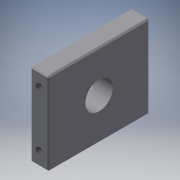
# Autodesk Inventor part: Ramka4
Saved by Autodesk Inventor 2019 (Build 230136000, 136)
## iProperties
Created: 2020-08-21
Part Number: Ramka4
Material: Steel(1)
Document SubType Name: Modeling
Designer: estee
Density: 7.85 g/cm^3
Appearance: Plate(1)
Author: estee
Autodesk Inventor part; units mm, degrees
ref_plane "YZ Plane" through (0, 0, 0) normal (1, 0, 0) x (0, 1, 0)
ref_plane "XZ Plane" through (0, 0, 0) normal (0, 1, 0) x (-1, 0, 0)
ref_plane "XY Plane" through (0, 0, 0) normal (0, 0, 1) x (1, 0, 0)
sketch "Sketch1" plane through (0, 0, 0) normal (1, 0, 0) x (0, 1, 0)
  line L0 (0, 0) -> (-18, 0)
  line L1 (-18, 0) -> (-18, -22)
  line L2 (-18, -22) -> (0, -22)
  line L3 (0, -22) -> (0, 0)
  dimension "d0" = 18
  dimension "d1" = 22
  constraints: 8 end point, 2 parallel, 1 horizontal, 1 perpendicular
  measures "d0" distance of L2.end L1.end
  measures "d1" distance of L2.end L0.start
extrude "Extrusion1" add sketch "Sketch1" along normal blind 4
chamfer "Chamfer1" distance 0.3 angle 45 12 edges at (4, 0, -11) (0, 0, -11) (2, 0, -22) (4, -9, 0) (2, 0, 0) (0, -9, -22) (2, -18, -22) (4, -9, -22) (4, -18, -11) (0, -18, -11) (0, -9, 0) (2, -18, 0)
sketch "Sketch2" plane through (0.3, -17.7, 0) normal (0, 0, 1) x (1, 0, 0)
  line L0 (-0.3, 17.4) -> (-0.3, 0) projected
  line L1 (3.4, 17.7) -> (0, 17.7) projected
  line L2 (0, -0.3) -> (3.4, -0.3) projected
  point P0 (-0.3, 17.7)
  point P1 (1.7, 14.7)
  point P2 (1.7, 2.7)
  dimension "d7" = 2
  dimension "d8" = 2
  dimension "d9" = 3
  dimension "d10" = 3
  measures "d7" distance from line of L0 point (1.7, 14.7)
  measures "d8" distance from line of L0 point (1.7, 2.7)
  measures "d9" distance from line of L1 point (1.7, 14.7)
  measures "d10" distance from line of L2 point (1.7, 2.7)
hole "Hole1" at (2, -3, 0) at (2, -15, 0) direction (0, 0, -1) diameter 1.567 depth 6.3 tip angle 118 thread size "M2x0.4" class "6H" standard "ISO Metric profile"
sketch "Sketch3" plane through (3.7, -17.7, -22) normal (0, 0, -1) x (-1, 0, 0)
  circle A0 centre (1.7, 2.7) radius 0.7835 projected
  circle A1 centre (1.7, 14.7) radius 0.7835 projected
  point P0 (3.7, 17.7)
  point P1 (1.7, 2.7)
  point P2 (1.7, 14.7)
  constraints: 2 coincident
hole "Hole2" at (2, -15, -22) at (2, -3, -22) direction (0, 0, 1) diameter 1.567 depth 6.3 tip angle 118 thread size "M2x0.4" class "6H" standard "ISO Metric profile"
sketch "Sketch4" plane through (0, 0, 0) normal (-1, 0, 0) x (0, 0, 1)
  line L0 (-22, -0.3) -> (-22, -17.7) projected
  line L1 (-0.3, 0) -> (-21.7, 0) projected
  point P0 (0, 0)
  point P1 (-11, -9)
  dimension "d25" = 11
  dimension "d26" = 9
  measures "d25" distance from line of L0 point (-11, -9)
  measures "d26" distance from line of L1 point (-11, -9)
hole "Hole3" at (0, -9, -11) direction (1, 0, 0) diameter 4 depth 6.3 tip angle 118
body "Solid1"
